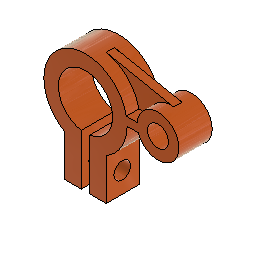
Design 8 v1 (Autodesk Fusion 360 design; units mm, degrees)
Autodesk Fusion 360 part; units mm, degrees
sketch "Sketch1" plane through (0, 0, 0) normal (0, 1, 0) x (1, 0, 0)
  line L0 (0, 0) -> (0, -1175.3412)
  line L1 (0, -1175.3412) -> (0, 325) construction
  line L2 (0, 0) -> (-1356.5029, 0) construction
  circle A0 centre (871.6879, -79.2241) radius 125
  circle A1 centre (871.6879, -79.2241) radius 250
  line L3 (-50, 255) -> (50, 255)
  line L4 (50, 321.1308) -> (50, 933.0127)
  line L5 (-50, 945) -> (-50, 255)
  line L6 (250, 433.0127) -> (250, 933.0127)
  line L7 (-250, 933.0127) -> (-250, 433.0127)
  line L8 (635.6485, 3.1495) -> (499.9901, 3.1495)
  line L9 (490.5883, -96.5563) -> (622.2894, -96.5563)
  line L10 (-1356.5029, 0) -> (466.5356, 0) construction
  line L11 (634.5728, 0) -> (675.4964, 0) construction
  line L12 (775, 0) -> (1559.7574, 0) construction
  line L13 (250, 933.0127) -> (48.2627, 933.0127)
  line L14 (-48.2627, 933.0127) -> (-250, 933.0127)
  line L15 (-48.2627, 933.0127) -> (-50, 945) construction
  arc A2 (-250, 433.0127) -> (250, 433.0127) centre (0, 0) ccw
  arc A3 (-50, 321.1308) -> (50, 321.1308) centre (0, 0) ccw
  line L16 (99.0099, -490.099) -> (909.823, -326.2984)
  dimension "d1" = 650
  dimension "d2" = 1000
  dimension "d3" = 250
  dimension "d4" = 500
  dimension "d7" = 500
  dimension "d8" = 500
  dimension "d9" = 933.0127
  constraint coincident L0.start L2.start
  constraint vertical L0
  constraint parallel L0 L1
  constraint perpendicular L0 L2
  constraint perpendicular L0 L10
  constraint concentric A0 A1
  constraint horizontal L3
  constraint perpendicular L3 L4
  constraint parallel L4 L5
  constraint vertical L6
  constraint horizontal L13
  constraint vertical L7
  constraint horizontal L8
  constraint parallel L8 L9
  constraint coincident L9.start A2
  constraint collinear L10 L11
  constraint coincident L8.end A2
  constraint coincident A1 L8.start
  constraint coincident A0 L12.start
  constraint collinear L11 L12
  constraint coincident A1 L9.end
  constraint collinear L13 L14
  constraint coincident L13 L4.end
  constraint coincident L5 A3.start
  constraint coincident A1 L11.start
  constraint coincident A1 L16.end
  constraint tangent A2 L16
  constraint coincident A2 L16.start
  measures "d1" diameter of A3
  measures "d2" diameter of A2
  measures "d3" diameter of A0
  measures "d4" diameter of A1
  measures "d7" distance of L7.end L6.start
  measures "d8" distance of L7.end L7.start
  measures "d9" distance of L0.start L13
extrude "Extrude1" add sketch "Sketch1" along normal mid plane 400 contours L0 L4 L6 L13 A2 A3 | L0 L5 L7 L14 A2 A3 | A1 L8 L9 A2 | A1
extrude "Extrude2" add sketch "Sketch1" along normal mid plane 100 contours A1 L9 A2 L16
hole "Hole1" at (250, -9.09, -683.0127) direction (-1, 0, 0) diameter 200 end through all
